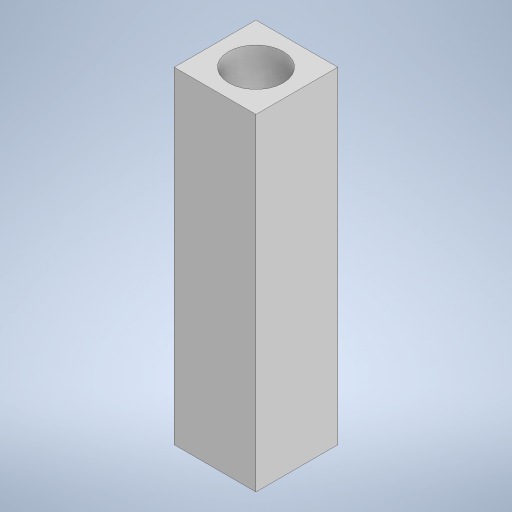
# Autodesk Inventor part: ArduinoStilts
Saved by Autodesk Inventor 2023 (Build 270158000, 158)
## iProperties
Created: 2023-09-26
Part Number: ArduinoStilts
Material: Generic
Document SubType Name: Modeling
Designer: Gage
Density: 1 g/cm^3
Appearance: Default
Author: Gage
Autodesk Inventor part; units mm, degrees
ref_plane "YZ Plane" through (0, 0, 0) normal (1, 0, 0) x (0, 1, 0)
ref_plane "XZ Plane" through (0, 0, 0) normal (0, 1, 0) x (-1, 0, 0)
ref_plane "XY Plane" through (0, 0, 0) normal (0, 0, 1) x (1, 0, 0)
sketch "Sketch1" plane through (0, 0, 0) normal (0, 0, 1) x (1, 0, 0)
  line L0 (-2.3813, 9.525) -> (2.3813, 9.525)
  line L1 (2.3813, 9.525) -> (2.3813, -9.525)
  line L2 (2.3813, -9.525) -> (-2.3813, -9.525)
  line L3 (-2.3813, -9.525) -> (-2.3813, 9.525)
  point P0 (0, 0)
  point P1 (2.3813, 0)
  point P2 (0, 9.525)
  dimension "d0" = 4.7625
  dimension "d1" = 19.05
  constraints: 8 end point, 2 midpoint, 2 parallel, 1 horizontal, 1 horizontal alignment, 1 perpendicular, 1 vertical alignment
  measures "d0" distance of L1.end L2.end
  measures "d1" distance of L0.end L1.end
extrude "Extrusion1" add sketch "Sketch1" along normal blind 4.7625
sketch "Sketch2" plane through (-2.3813, 9.525, 0) normal (0, 1, 0) x (1, 0, 0)
  circle A0 centre (2.3813, -2.3813) radius 1.5875
  line L0 (0, 0) -> (0, -4.7625) projected
  line L1 (4.7625, -4.7625) -> (0, -4.7625) projected
  line L2 (4.7625, 0) -> (0, 0) projected
  line L3 (4.7625, 0) -> (4.7625, -4.7625) projected
  point P0 (2.3813, 0)
  dimension "d4" = 3.175
  dimension "d9" = 2.3813
  dimension "d10" = 2.3813
  constraints: 1 centre point
  measures "d4" diameter of A0
  measures "d9" distance from line of L2 A0.centre
  measures "d10" distance from line of L3 A0.centre
extrude "Extrusion2" cut sketch "Sketch2" against normal through all contours A0
body "Solid1"
